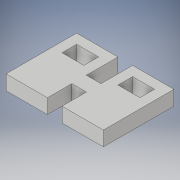
# Autodesk Inventor part: flipper-holder
Saved by Autodesk Inventor 2017 (Build 210142000, 142)
## iProperties
Created: 2017-03-03
Part Number: flipper-holder
Material: Generic
Document SubType Name: Modeling
Designer: John
Density: 1 g/cm^3
Appearance: Default
Author: John
Autodesk Inventor part; units mm, degrees
ref_plane "YZ Plane" through (0, 0, 0) normal (1, 0, 0) x (0, 1, 0)
ref_plane "XZ Plane" through (0, 0, 0) normal (0, 1, 0) x (-1, 0, 0)
ref_plane "XY Plane" through (0, 0, 0) normal (0, 0, 1) x (1, 0, 0)
sketch "Sketch1" plane through (0, 0, 0) normal (0, 1, 0) x (-1, 0, 0)
  line L0 (4.7584, -0.779) -> (21.7584, -0.779)
  line L1 (21.7584, -0.779) -> (21.7584, -13.779)
  line L2 (21.7584, -13.779) -> (4.7584, -13.779)
  line L3 (4.7584, -13.779) -> (4.7584, -0.779)
  line L4 (8.7584, -3.779) -> (17.7584, -3.779)
  line L5 (17.7584, -3.779) -> (17.7584, -9.779)
  line L6 (17.7584, -9.779) -> (8.7584, -9.779)
  line L7 (8.7584, -9.779) -> (8.7584, -3.779)
  line L8 (21.7584, -0.779) -> (-18.2416, -0.779)
  line L9 (-18.2416, -0.779) -> (-18.2416, 5.221)
  line L10 (-18.2416, 5.221) -> (21.7584, 5.221)
  line L11 (21.7584, 5.221) -> (21.7584, -0.779)
  line L12 (17.7584, -6.6245) -> (21.7584, -6.6245) construction
  line L13 (8.7584, -6.779) -> (4.7584, -6.779) construction
  line L14 (-18.2416, -0.779) -> (-1.2416, -0.779)
  line L15 (-1.2416, -0.779) -> (-1.2416, -13.779)
  line L16 (-1.2416, -13.779) -> (-18.2416, -13.779)
  line L17 (-18.2416, -13.779) -> (-18.2416, -0.779)
  line L18 (-14.2416, -3.779) -> (-5.2416, -3.779)
  line L19 (-5.2416, -3.779) -> (-5.2416, -9.779)
  line L20 (-5.2416, -9.779) -> (-14.2416, -9.779)
  line L21 (-14.2416, -9.779) -> (-14.2416, -3.779)
  line L22 (-5.2416, -6.779) -> (-1.2416, -6.779) construction
  line L23 (-18.2416, -6.779) -> (-14.2416, -6.779) construction
  line L24 (21.7584, 5.221) -> (4.7584, 5.221)
  line L25 (4.7584, 5.221) -> (4.7584, 15.221)
  line L26 (4.7584, 15.221) -> (21.7584, 15.221)
  line L27 (21.7584, 15.221) -> (21.7584, 5.221)
  line L28 (-18.2416, 5.221) -> (-1.2416, 5.221)
  line L29 (-1.2416, 5.221) -> (-1.2416, 15.221)
  line L30 (-1.2416, 15.221) -> (-18.2416, 15.221)
  line L31 (-18.2416, 15.221) -> (-18.2416, 5.221)
  point P0 (0, 0)
  dimension "d0" = 9
  dimension "d1" = 6
  dimension "d2" = 4
  dimension "d3" = 40
  dimension "d4" = 6
  dimension "d5" = 4
  dimension "d6" = 3
  dimension "d7" = 4
  dimension "d8" = 9
  dimension "d9" = 6
  dimension "d10" = 3
  dimension "d11" = 4
  dimension "d14" = 10
  dimension "d15" = 10
  constraints: 64 end point, 14 parallel, 10 perpendicular, 7 horizontal, 6 point on line, 3 midpoint, 2 equal length
  measures "d0" distance of L5.end L6.end
  measures "d1" distance of L4.end L5.end
  measures "d2" distance between parallel lines of L2 L6
  measures "d3" distance of L9.end L10.end
  measures "d4" distance of L8.end L9.end
  measures "d5" distance of L12.start L12.end
  measures "d6" distance between parallel lines of L4 L8
  measures "d7" distance between parallel lines of L16 L20
  measures "d8" distance of L19.end L20.end
  measures "d9" distance of L18.end L19.end
  measures "d10" distance between parallel lines of L8 L18
  measures "d11" distance of L22.start L22.end
  measures "d14" distance of L30.end L9.end
  measures "d15" distance of L24.end L25.end
extrude "Extrusion1" add sketch "Sketch1" along normal blind 6
equation "\"d5\" = d2"
equation "\"d7\" = d2"
equation "\"d8\" = d0"
equation "\"d9\" = d1"
equation "\"d10\" = d6"
equation "\"d11\" = d5"
equation "\"d15\" = d14"
body "Solid1"
